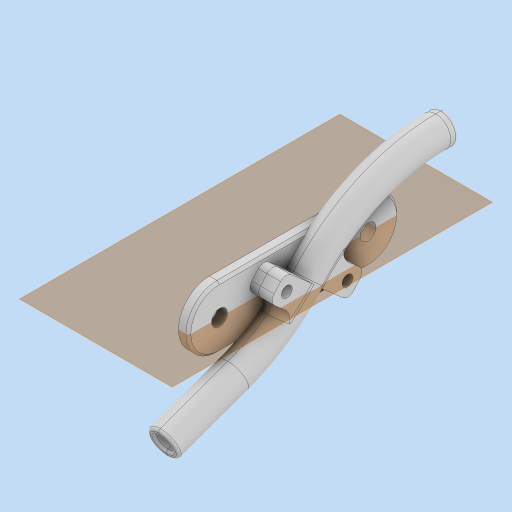
# Autodesk Inventor part: HF-Kabeldurchführung-BackPanel-Multibody
Saved by Autodesk Inventor 2023.2 (Build 272271000, 271)
## iProperties
Created: 2024-01-10
Part Number: HF-Kabeldurchführung-BackPanel-Multibody
Material: Generisch
Document SubType Name: Modeling
Designer: Nils Bade
Density: 1 g/cm^3
Appearance: Vorgabe
Author: Nils Bade
Autodesk Inventor part; units mm, degrees
ref_plane "YZ Plane" through (0, 0, 0) normal (1, 0, 0) x (0, 1, 0)
sketch "T-SLOT 4040" plane through (0, 0, 0) normal (0, 0, 1) x (1, 0, 0)
  line L0 (-20, -20) -> (20, -20)
  line L1 (20, -20) -> (20, -5)
  line L2 (20, 20) -> (-20, 20)
  line L3 (-20, 20) -> (-20, -20)
  line L4 (-20, -20) -> (20, 20) construction
  line L5 (20, -20) -> (-20, 20) construction
  line L6 (20, 5) -> (12, 5)
  line L7 (12, 5) -> (12, -5)
  line L8 (12, -5) -> (20, -5)
  line L9 (20, -5) -> (20, 5) construction
  line L10 (20, 5) -> (20, 20)
  line L11 (20, -5) -> (20, 5) construction
  point P0 (0, 0)
  point P1 (20, 0)
  dimension "d0" = 40
  dimension "d1" = 40
  dimension "d2" = 8
  dimension "d3" = 10
  constraints: 24 end point, 6 parallel, 4 perpendicular, 3 midpoint, 2 horizontal
  measures "d0" distance of L2.end L2.start
  measures "d1" distance of L2.start L0.end
  measures "d2" distance of L1.end L7.end
  measures "d3" distance of L7.end L6.end
surface extrude "Extrusionsfläche1" sketch "T-SLOT 4040" along normal mid plane 100 shown yes curves L3 L0 L1 L8 L7 L6 L10 L2
ref_plane "Anschlussebene" through (0, -20, 40) normal (0, -0.3420201, 0.9396926) x (-1, 0, 0)
ref_plane "Kabelebene" through (27.5, -20, -50) normal (-1, 0, 0) x (0, 0, 1)
sketch "S-KabelSpline" plane through (27.5, -20, -50) normal (-1, 0, 0) x (0, 0, 1)
  line L0 (123.1673, 91.1265) -> (62.0655, -76.7493) construction
  line L1 (0, 0) -> (100, 0) construction
  line L2 (0, 0) -> (100, 0) construction
  line L3 (90, 0) -> (87.6007, 0.8733)
  arc A0 (58.6272, 20.8259) -> (87.6007, 0.8733) centre (111.5421, 66.6518) ccw
  arc A1 (58.6272, 20.8259) -> (5.7122, 45) centre (5.7122, -25) ccw
  line L4 (2.7076, 45) -> (5.7122, 45)
  line L5 (90, 0) -> (115.7914, -9.3873)
  line L6 (0, 40) -> (100, 40) construction
  point P0 (50, 20)
  dimension "d9" = 70
  dimension "d10" = 70
  dimension "d11" = 30
  dimension "d12" = 5
  constraints: 6 end point, 4 point on circle, 3 tangent, 2 centre point, 2 perpendicular, 2 point on line, 1 horizontal
  measures "d9" radius of A0
  measures "d10" radius of A1
  measures "d11" distance of L5.end L3.end
  measures "d12" distance between parallel lines of L6 L4
sketch "S-Führungsquerschnitt" plane through (0, -20, 40) normal (0, -0.3420201, 0.9396926) x (-1, 0, 0)
  line L0 (-42, 0) -> (7, 0) projected
  line L1 (-27.5, -96.9747) -> (-27.5, 81.6749) construction
  circle A0 centre (-27.5, 0) radius 6
  point P0 (0, -5.113)
  dimension "d13" = 12
  constraints: 1 centre point, 1 coincident
  measures "d13" diameter of A0
sweep "Sweeping1" add profiles "S-Führungsquerschnitt" path "S-KabelSpline" path curves L5 L3 A0 A1 L4
sketch "S-Base" plane through (20, -20, -50) normal (-1, 0, 0) x (0, 0, 1)
  line L0 (29.5424, 20) -> (89.5424, 20) construction
  line L1 (29.5424, 7.5) -> (89.5424, 7.5)
  line L2 (89.5424, 32.5) -> (29.5424, 32.5)
  arc A0 (29.5424, 32.5) -> (29.5424, 7.5) centre (29.5424, 20) ccw
  arc A1 (89.5424, 7.5) -> (89.5424, 32.5) centre (89.5424, 20) ccw
  line L3 (-20.4222, 20) -> (141.4864, 20) construction
  circle A2 centre (89.5424, 20) radius 3.15
  circle A3 centre (89.5424, 20) radius 5 construction
  line L4 (0, 25) -> (100, 25) construction
  line L5 (0, 15) -> (100, 15) construction
  line L6 (59.5424, 32.5) -> (59.5424, 7.5) construction
  circle A4 centre (29.5424, 20) radius 3.15
  circle A5 centre (29.5424, 20) radius 5 construction
  line L7 (0, 25) -> (100, 25) projected
  line L8 (79.5424, 15) -> (39.5424, 15) construction
  line L9 (39.5424, 15) -> (39.5424, 25) construction
  line L10 (39.5424, 25) -> (79.5424, 25) construction
  line L11 (79.5424, 25) -> (79.5424, 15) construction
  line L12 (39.6424, 24.9) -> (39.6424, 15.1)
  line L13 (39.6424, 15.1) -> (79.4424, 15.1)
  line L14 (79.4424, 15.1) -> (79.4424, 24.9)
  line L15 (79.4424, 24.9) -> (39.6424, 24.9)
  point P0 (59.5424, 20)
  dimension "d16" = 30
  dimension "d17" = 25
  dimension "d18" = 6.3
  dimension "d19" = 10
  dimension "d21" = 20
  dimension "d22" = 0.1
  constraints: 26 end point, 6 centre point, 5 parallel, 4 point on circle, 4 tangent, 3 coincident, 3 midpoint, 2 horizontal, 2 perpendicular, 2 point on line, 2 symmetric about line, 1 collinear, 6 other
  measures "d16" distance of point (59.542, 20) L0.end
  measures "d17" diameter of A1
  measures "d18" diameter of A2
  measures "d19" diameter of A3
  measures "d21" distance between parallel lines of L6 L9
  measures "d22" distance between parallel lines of L9 L12
extrude "Ex-Base1" add sketch "S-Base" against normal blind 4 contours A0 L2 A1 L1 | L15 L14 L13 L12
extrude "Ex-Base-Schiene" add sketch "S-Base" along normal blind 2.5 contours L15 L14 L13 L12
ref_plane "FlanschSkizzenEbene" through (24, -20, -50) normal (1, 0, 0) x (0, 0, -1)
sketch "S-Pressflansche" plane through (24, -20, -50) normal (1, 0, 0) x (0, 0, -1)
  line L0 (-54.0916, 16.898) -> (-63.1627, 24.7538) construction
  line L1 (-58.6272, 20.8259) -> (-0.9589, 87.4152) construction
  line L2 (-58.6272, 20.8259) -> (-116.2954, -45.7634) construction
  line L3 (-65.5678, 12.8116) -> (-59.0212, 20.3709)
  line L4 (-59.0212, 20.3709) -> (-71.872, 31.5)
  line L5 (-71.872, 31.5) -> (-78.4185, 23.9407)
  line L6 (-78.4185, 23.9407) -> (-65.5678, 12.8116)
  line L7 (-74.6389, 20.6674) -> (-68.0924, 28.2267) construction
  circle A0 centre (-71.3656, 24.4471) radius 2.15
  circle A1 centre (-71.3656, 24.4471) radius 3.5 construction
  line L8 (-67.1135, 23.6288) -> (-69.9483, 20.3555)
  line L9 (-69.9483, 20.3555) -> (-74.2004, 21.1738)
  line L10 (-74.2004, 21.1738) -> (-75.6177, 25.2654)
  line L11 (-75.6177, 25.2654) -> (-72.783, 28.5387)
  line L12 (-72.783, 28.5387) -> (-68.5309, 27.7203)
  line L13 (-68.5309, 27.7203) -> (-67.1135, 23.6288)
  line L14 (-59.0212, 20.3709) -> (-46.1705, 9.2417) construction
  line L15 (-46.1705, 9.2417) -> (-52.717, 1.6824) construction
  line L16 (-52.717, 1.6824) -> (-65.5678, 12.8116) construction
  line L17 (-56.4966, 4.9557) -> (-49.9501, 12.515) construction
  circle A2 centre (-53.2234, 8.7354) radius 2.15 construction
  circle A3 centre (-53.2234, 8.7354) radius 3.5 construction
  line L18 (-54.6407, 12.8269) -> (-57.4755, 9.5537) construction
  line L19 (-57.4755, 9.5537) -> (-56.0581, 5.4621) construction
  line L20 (-56.0581, 5.4621) -> (-51.806, 4.6438) construction
  line L21 (-51.806, 4.6438) -> (-48.9713, 7.917) construction
  line L22 (-48.9713, 7.917) -> (-50.3886, 12.0086) construction
  line L23 (-50.3886, 12.0086) -> (-54.6407, 12.8269) construction
  line L24 (-51.1253, 16.8862) -> (-49.708, 12.7946)
  line L25 (-48.2906, 20.1594) -> (-51.1253, 16.8862)
  line L26 (-52.6711, 27.7034) -> (-39.8203, 16.5742)
  line L27 (-46.3669, 9.0149) -> (-59.2176, 20.1441)
  line L28 (-49.708, 12.7946) -> (-45.4559, 11.9763)
  line L29 (-44.0385, 19.3411) -> (-48.2906, 20.1594)
  circle A4 centre (-46.8732, 16.0678) radius 2.15
  circle A5 centre (-46.8732, 16.0678) radius 3.5 construction
  line L30 (-50.1465, 12.2882) -> (-43.5999, 19.8475) construction
  line L31 (-45.4559, 11.9763) -> (-42.6211, 15.2495)
  line L32 (-42.6211, 15.2495) -> (-44.0385, 19.3411)
  line L33 (-39.8203, 16.5742) -> (-46.3669, 9.0149)
  line L34 (-53.6682, 32.5) -> (-89.5424, 32.5) projected
  line L35 (-52.6711, 27.7034) -> (-59.2176, 20.1441)
  point P0 (-50, 20)
  point P1 (-54.9432, 17.6355)
  dimension "d28" = 10
  dimension "d29" = 17
  dimension "d30" = 4.3
  dimension "d31" = 7
  dimension "d32" = 7.5
  dimension "d33" = 5
  dimension "d36" = 9.7
  dimension "d41" = 1
  constraints: 68 end point, 14 symmetric about line, 8 point on line, 6 centre point, 6 coincident, 3 parallel, 3 perpendicular, 2 midpoint, 1 collinear, 43 other
  measures "d28" distance of L4.end L5.end
  measures "d29" distance of L3.end L4.end
  measures "d30" diameter of A0
  measures "d31" diameter of A1
  measures "d32" distance between parallel lines of L10 L13
  measures "d33" distance between parallel lines of L5 L7
  measures "d36" distance of L19.start L24.start
  measures "d41" distance from line of L34 L4.end
extrude "Ex-Pressflansche1" add sketch "S-Pressflansche" along normal blind 9 contours L6 L5 L4 L3 | L3 L35 L26 L33 L27 | A0 | L8 L9 L10 L11 L12 L13 | L25 L29 L32 L31 L28 L24 | A4
extrude "Ex-Pressflansche2-Bohrungen" cut sketch "S-Pressflansche" along normal blind 15 and the other way blind 10 contours A0 | A4
extrude "Ex-Pressflansche3-Muttern" cut sketch "S-Pressflansche" along normal blind 1 and the other way blind 10 contours A0 | L8 L9 L10 L11 L12 L13 | L25 L29 L32 L31 L28 L24 | A4
sketch "S-Kabeldurchmesser" plane through (27.5, -29.3873, 65.7914) normal (0, -0.3420201, 0.9396926) x (1, 0, 0)
  circle A0 centre (0, 0) radius 6 projected
  circle A1 centre (0, 0) radius 3.25
  circle A2 centre (0, 0) radius 2.25
  point P0 (-27.5, 5.113)
  dimension "d52" = 6.5
  dimension "d53" = 4.5
  constraints: 2 centre point, 2 coincident
  measures "d52" diameter of A1
  measures "d53" diameter of A2
sweep "Sweeping2" cut profiles "S-Kabeldurchmesser" path "S-KabelSpline" path curves L5 L3 A0 A1 L4 contours A2
extrude "Extrusion6" cut sketch "S-Kabeldurchmesser" against normal blind 30 contours A1
fillet "Rundung-3mm" radius 3 8 edges at (28.5, -10.9851, -3.6331) (28.5, -3.4258, -10.1797) (29.0995, 3.4935, -2.19) (29.1025, -2.8263, 20.6047) (28.5, 11.5, 21.872) (28.5, 3.9407, 28.4185) (33, 2.6019, 3.7133) (33, -1.6976, 14.294)
fillet "Rundung-1mm" radius 1 4 edges at (25.25, 25, -47.2924) (33.5, 25, -47.2924) (24.25, -29.3873, 65.7914) (33.5, -29.3873, 65.7914)
chamfer "Fase-1mm" distance 1 angle 45 12 edges at (17.5, -4.9, 14.9745) (17.5, 0, 29.4424) (17.5, 4.9, 27.4668) (17.5, 4.9, 3.5981) (17.5, 0, -10.3576) (17.5, -4.9, -8.8035) (24, 0, -32.9576) (24, 12.5, -17.082) (24, -12.5, -2.4093) (24, 12.5, 21.6053) (24, 0, 52.0424) (24, -12.5, 36.9174)
split body "Trennen1" result two bodies by plane through (27.5, -20, -50) normal (-1, 0, 0) first body at (20.5, -11.0079, 4.8469)
ref_plane "XY-VersatzEbene" through (0, 0, 40) normal (0, 0, 1) x (1, 0, 0)
